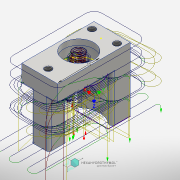
# Autodesk Inventor part: cam-flying-mount-rev2
Saved by Autodesk Inventor 2016 (Build 200138000, 138)
## iProperties
Created: 2015-05-15
Part Number: cam-flying-mount-rev2
Material: Aluminum 6061
Document SubType Name: Modeling
Designer: as
Mass: 7.99147 g
Surface Area: 27.6223 cm^2
Volume: 2.95981 cm^3
Density: 2.7 g/cm^3
Appearance: Aluminum - Flat
Author: as
Autodesk Inventor part; units mm, degrees
ref_plane "YZ Plane" through (0, 0, 0) normal (1, 0, 0) x (0, 1, 0)
ref_plane "XZ Plane" through (0, 0, 0) normal (0, 1, 0) x (-1, 0, 0)
ref_plane "XY Plane" through (0, 0, 0) normal (0, 0, 1) x (1, 0, 0)
sketch "Sketch1" plane through (0, 0, 0) normal (0, 0, 1) x (1, 0, 0)
  line L0 (-6.5, 4) -> (6.5, 4)
  line L1 (6.5, 4) -> (6.5, -4)
  line L2 (6.5, -4) -> (-6.5, -4)
  line L3 (-6.5, -4) -> (-6.5, 4)
  line L4 (-6.5, 4) -> (6.5, -4) construction
  line L5 (6.5, 4) -> (-6.5, -4) construction
  point P0 (0, 0)
  point P1 (4.5, 1.25)
  point P2 (-4.5, 1.25)
  dimension "d0" = 13
  dimension "d1" = 8
  dimension "d64" = 2.75
  dimension "d65" = 2
  dimension "d66" = 2.75
  dimension "d67" = 2
  constraints: 12 end point, 2 midpoint, 2 parallel, 1 horizontal, 1 perpendicular
  measures "d0" distance of L1.end L2.end
  measures "d1" distance of L0.end L1.end
  measures "d64" distance from line of point (-4.5, 1.25) L0
  measures "d65" distance from line of L3 point (-4.5, 1.25)
  measures "d66" distance from line of L0 point (4.5, 1.25)
  measures "d67" distance from line of point (4.5, 1.25) L1
extrude "Extrusion1" add sketch "Sketch1" along normal blind 48
hole "Hole1" at (-4.5, 1.25, 0) at (4.5, 1.25, 0) direction (0, 0, 1) diameter 2.459 end through all thread size "M3x0.5" class "6H" standard "ISO Metric profile"
sketch "Sketch6" plane through (-6.5, -4, 0) normal (0, -1, 0) x (1, 0, 0)
  line L0 (0.2, 0) -> (0, 0) projected
  line L1 (12.8, 0) -> (12.8, 36.9748) projected
  line L2 (0, 0) -> (12.8, 0)
  line L3 (12.8, 0) -> (12.8, 17)
  line L4 (12.8, 17) -> (0, 17)
  line L5 (0, 17) -> (0, 0)
  line L6 (13, 0) -> (13, 48) projected
  line L7 (0, 17) -> (13, 17)
  line L8 (13, 17) -> (13, 23)
  line L9 (13, 23) -> (0, 23)
  line L10 (0, 23) -> (0, 17)
  point P0 (6.5, 0)
  point P1 (12.8, 36.8338)
  point P2 (13, 36.8338)
  point P3 (13, 37.0101)
  dimension "d60" = 17
  dimension "d61" = 6
  constraints: 16 end point, 4 parallel, 2 horizontal, 2 perpendicular, 2 point on line
  measures "d60" distance of L3.end L2.end
  measures "d61" distance of L8.end L7.end
extrude "Extrusion3" add sketch "Sketch6" along normal blind 18 contours L10 L9 L1 L4 | L1 L9 L6 L7
sketch "Sketch7" plane through (6.5, -4, 17) normal (0, 0, -1) x (-1, 0, 0)
  line L0 (13, 8) -> (0, 8) projected
  circle A0 centre (6.5, -4) radius 6
  point P0 (6.5, 4)
  dimension "d68" = 12
  dimension "d69" = 12
  constraints: 1 centre point
  measures "d68" diameter of A0
  measures "d69" distance from line of L0 A0.centre
extrude "Extrusion4" cut sketch "Sketch7" against normal blind 4
sketch "Sketch8" plane through (6.5, -22, 17) normal (0, 0, -1) x (-1, 0, 0)
  circle A0 centre (6.5, 14) radius 6 projected
  circle A1 centre (6.5, 14) radius 7.5
  point P0 (6.5, 22)
  dimension "d72" = 15
  constraints: 1 centre point, 1 coincident
  measures "d72" diameter of A1
extrude "Extrusion5" cut sketch "Sketch8" along normal through all contours A0 | A1
sketch "Sketch9" plane through (0, -8, 21) normal (0, 0, -1) x (-1, 0, 0)
  circle A0 centre (0, 0) radius 5.4
  point P0 (0, 8)
  dimension "d75" = 10.8
  constraints: 1 centre point
  measures "d75" diameter of A0
extrude "Extrusion6" cut sketch "Sketch9" against normal up to surface (2 mm away)
sketch "Sketch10" plane through (6.5, -22, 17) normal (0, 0, -1) x (-1, 0, 0)
  line L0 (3.25, 6.5) -> (3.25, 0)
  line L1 (3.25, 0) -> (9.75, 0)
  line L2 (9.75, 0) -> (9.75, 6.5)
  line L3 (9.75, 6.5) -> (3.25, 6.5)
  line L4 (3.25, 6.5) -> (9.75, 0) construction
  line L5 (3.25, 0) -> (9.75, 6.5) construction
  circle A0 centre (6.5, 14) radius 6 projected
  circle A1 centre (6.5, 14) radius 7.5 projected
  point P0 (6.5, 22)
  point P1 (6.5, 3.25)
  dimension "d78" = 6.5
  dimension "d80" = 6.5
  dimension "d81" = 3.25
  dimension "d95" = 7.5
  constraints: 12 end point, 2 midpoint, 2 parallel, 1 horizontal, 1 perpendicular
  measures "d78" distance of L1.end L0.end
  measures "d80" distance of L1.end L2.end
  measures "d81" distance from line of point (6.5, 22) L2
  measures "d95" distance from line of L3 A1.centre
extrude "Extrusion7" add sketch "Sketch10" along normal up to surface (17 mm away) contours L3 L2 L1 L0
sketch "Sketch11" plane through (3.25, -15.5, 0) normal (0, 0, -1) x (-1, 0, 0)
  line L0 (9.75, 19.5) -> (-3.25, 19.5) projected
  line L1 (-3.25, 19.5) -> (-3.25, 11.5) projected
  line L2 (6.5, 0) -> (0, 0) projected
  point P0 (3.25, 15.5)
  point P1 (3.25, -3.5)
  point P2 (9.55, 19.5)
  point P3 (-3.05, 19.5)
  point P4 (-3.25, 19.3)
  dimension "d85" = 6.5
  dimension "d96" = 3.5
  dimension "d97" = 23
  measures "d85" distance from line of L1 point (3.25, -3.5)
  measures "d96" distance from line of L2 point (3.25, -3.5)
  measures "d97" distance from line of point (3.25, -3.5) L0
hole "Hole5" at (0, -19, 0) direction (0, 0, 1) diameter 2.459 end through all thread size "M3x0.5" class "6H" standard "ISO Metric profile"
fillet "Fillet2" radius 1 8 edges at (-6.3443, -4, 8.5) (6.3443, -4, 8.5) (-6.5, -4, 8.5) (6.5, -4, 8.5) (-3.25, -15.5, 8.5) (3.25, -15.5, 8.5) (3.25, -22, 8.5) (-3.25, -22, 8.5)
sketch "Sketch13" plane through (0, 0, 0) normal (0, 0, -1) x (-1, 0, 0)
  point P0 (-4.5, 1.25)
move faces "Move1" translate (0, 0, -25) faces at (-1.2282, -2.5568, 48)
sketch "Sketch15" plane through (-6.5, -22, 23) normal (0, 0, 1) x (1, 0, 0)
  point P0 (6.5, 22)
equation "\"d66\" = d64"
equation "\"d67\" = d65"
equation "\"d81\" = 0.5 * d78"
body "Solid1"
